Autodesk Fusion 360 part; units mm, degrees
(part 2 of 2)
sketch "Esquisse1" plane through (0, 0, 0) normal (0, 0, 1) x (1, 0, 0)
  circle A0 centre (0, 0) radius 40
  circle A1 centre (0, 0) radius 15
  line L0 (6, 3.4641) -> (0, 6.9282)
  line L1 (0, 6.9282) -> (-6, 3.4641)
  line L2 (-6, 3.4641) -> (-6, -3.4641)
  line L3 (-6, -3.4641) -> (0, -6.9282)
  line L4 (0, -6.9282) -> (6, -3.4641)
  line L5 (6, -3.4641) -> (6, 3.4641)
  circle A2 centre (40, 0) radius 5
  circle A3 centre (0, 0) radius 4.05
  dimension "d21" = 80
  dimension "d26" = 30
  dimension "d27" = 6
  dimension "d122" = 8.1
  constraint coincident A0.centre A1.centre
  constraint concentric A0 A1
  constraint coincident A0 A2.centre
  constraint concentric A1 A3
  measures "d21" diameter of A0
  measures "d26" diameter of A1
  measures "d27" distance of A0.centre L0
  measures "d122" diameter of A3
extrude "Extrusion1" add sketch "Esquisse1" along normal blind 6 contours A0 A2 picked at (28.6857, 8.6025)
extrude "Extrusion2" add sketch "Esquisse1" along normal blind 12 contours A1
extrude "Extrusion3" add sketch "Esquisse1" along normal blind 8 contours L0 L1 L2 L3 L4 L5
pattern_circular "Réseau C1" count 15 over 360 about axis through (0, 0, 0) along (0, 0, 1) of 1 faces at (39.2118, -4.9375, 4)

design "graduation_table_60_Z"
Autodesk Fusion 360 part; units mm, degrees
sketch "Esquisse1" plane through (0, 0, 0) normal (0, 0, 1) x (1, 0, 0)
  arc A0 (169.741, 98) -> (0, 196) centre (0, 0) ccw
  line L0 (0, 182) -> (13, 182)
  line L1 (16, 185) -> (16, 187.4887)
  line L2 (0, 196) -> (0, 193.2049)
  arc A1 (15.7439, 182.0039) -> (15.6111, 182.0119) centre (15.6954, 182.3046) ccw
  arc A2 (19.8621, 190.9699) -> (16, 187.4887) centre (19.5, 187.4887) ccw
  line L3 (0, 0) -> (215.5081, 124.4237) construction
  line L4 (191.1412, 0) -> (248.8473, 0) construction
  line L5 (169.741, 98) -> (157.6166, 91)
  line L6 (157.6166, 91) -> (156.1166, 93.5981)
  line L7 (157.2147, 97.6962) -> (160.0383, 99.3264)
  arc A3 (161.2274, 104.258) -> (19.8621, 190.9699) centre (0, 0) ccw
  line L8 (160.5038, 105.3686) -> (163.9734, 107.3718)
  line L9 (12, 195.6323) -> (12, 191.6246)
  line L10 (1.1843, 192.2221) -> (8, 193.5)
  line L11 (8, 193.5) -> (8, 184.5)
  line L12 (8, 184.5) -> (1.1843, 185.7779)
  line L13 (0, 184.7951) -> (0, 182)
  line L14 (0, 189) -> (13, 189) construction
  arc A4 (13, 182) -> (16, 185) centre (13, 185) ccw
  line L15 (0, 0) -> (0, 230) construction
  line L16 (162.5878, 96.3896) -> (168.6492, 85.891) construction
  line L17 (166.1037, 95.9) -> (170.8023, 90.5262)
  line L18 (170.6759, 89.764) -> (164.2817, 86.0724)
  line L19 (163.5585, 86.344) -> (161.2539, 93.1)
  line L20 (12, 195.6323) -> (12, 182)
  arc A5 (0, 193.2049) -> (1.1843, 192.2221) centre (1, 193.2049) ccw
  arc A6 (1.1843, 185.7779) -> (0, 184.7951) centre (1, 184.7951) ccw
  arc A7 (170.6759, 89.764) -> (170.8023, 90.5262) centre (170.4259, 90.1971) ccw
  arc A8 (163.5585, 86.344) -> (164.2817, 86.0724) centre (164.0317, 86.5054) ccw
  arc A9 (160.0383, 99.3264) -> (161.2274, 104.258) centre (158.2883, 102.3575) ccw
  arc A10 (157.2147, 97.6962) -> (156.1166, 93.5981) centre (158.7147, 95.0981) ccw
  point P0 (154.6166, 96.1962)
  point P1 (0, 192)
  point P2 (0, 186)
  point P3 (171.2027, 90.0682)
  point P4 (163.7549, 85.7682)
  dimension "d38" = 196
  dimension "d47" = 16
  dimension "d58" = 30
  dimension "d60" = 6
  dimension "d68" = 11
  dimension "d69" = 192
  dimension "d70" = 12
  dimension "d77" = 7
  dimension "d83" = 6
  dimension "d84" = 9
  dimension "d85" = 8
  dimension "d86" = 3
  dimension "d87" = 60
  dimension "d88" = 7
  dimension "d89" = 14
  dimension "d90" = 14
  dimension "d91" = 8.6
  dimension "d92" = 5.6
  dimension "d93" = 7.6
  dimension "d94" = 1
  dimension "d95" = 0.5
  dimension "d96" = 0.5
  dimension "d97" = 3.5
  dimension "d98" = 3
  dimension "d99" = 3.5
  constraint perpendicular L0 L1
  constraint tangent L0 A1
  constraint tangent L1 A1
  constraint tangent L1 A2
  constraint coincident A0.centre L3.start
  constraint coincident L3 A0.start
  constraint coincident L3 L5.end
  constraint perpendicular L3 L6
  constraint perpendicular L6 L7
  constraint coincident A3 L8.start
  constraint coincident A0 L8.end
  constraint parallel L3 L8
  constraint horizontal L0
  constraint coincident L2 A0.centre
  constraint coincident A0 L9.start
  constraint coincident A3 L9.end
  constraint vertical L9
  constraint coincident L2 P1
  constraint parallel L2 L11
  constraint perpendicular L0 L13
  constraint perpendicular L11 L14
  constraint symmetric L10 L12 L14
  constraint coincident P2 L13
  constraint tangent A2 A3
  constraint tangent L0 A4
  constraint tangent L1 A4
  constraint vertical L15
  constraint perpendicular L3 L16
  constraint coincident L3 L17.start
  constraint parallel L3 L18
  constraint coincident L5 L19.end
  constraint symmetric L16 L17 L19
  constraint coincident L0 L20.end
  constraint perpendicular L0 L20
  constraint coincident L14.start L2
  constraint coincident P1 L10
  constraint tangent L2 A5
  constraint tangent L10 A5
  constraint coincident P2 L12
  constraint coincident L14.start L13
  constraint tangent L12 A6
  constraint tangent L13 A6
  constraint equal A5 A6
  constraint coincident P3 L17
  constraint coincident P3 L18
  constraint tangent L17 A7
  constraint tangent L18 A7
  constraint coincident P4 L19
  constraint coincident P4 L18
  constraint tangent L19 A8
  constraint tangent L18 A8
  constraint tangent A3 A9
  constraint tangent L7 A9
  constraint coincident P0 L7
  constraint coincident P0 L6
  constraint tangent L7 A10
  constraint tangent L6 A10
  measures "d38" radius of A0
  measures "d47" distance of L1 L2
  measures "d58" angle of L3 L4
  measures "d60" distance of L5.end P0
  measures "d68" distance of L5 L8
  measures "d69" radius of A3
  measures "d70" distance of L2 L9
  measures "d77" distance of A0.end L14.start
  measures "d83" distance of P1 P2
  measures "d84" distance of L10.end L11.end
  measures "d85" distance of L11 L13
  measures "d86" radius of A4
  measures "d87" angle of L3 L15
  measures "d88" distance of A0.start L16
  measures "d89" distance of A0.end L0.start
  measures "d90" distance of A0.start L5.end
  measures "d91" distance of P3 P4
  measures "d92" distance of L17.start L19.end
  measures "d93" distance of L3 L18
  measures "d94" radius of A5
  measures "d95" radius of A7
  measures "d96" radius of A8
  measures "d97" radius of A9
  measures "d98" radius of A10
  measures "d99" radius of A2
extrude "Extrusion4" add sketch "Esquisse1" along normal blind 1.5
sketch "Esquisse3" plane through (0, 0, 0) normal (0, 0, 1) x (-1, 0, 0)
  arc A0 (-169.741, -98) -> (0, -196) centre (0, 0) ccw
  line L0 (0, -196) -> (0, -193.2049)
  line L1 (0, -182) -> (-13, -182)
  line L2 (-16, -185) -> (-16, -187.4887)
  arc A1 (-19.8621, -190.9699) -> (-16, -187.4887) centre (-19.5, -187.4887) ccw
  arc A2 (-161.2274, -104.258) -> (-19.8621, -190.9699) centre (0, 0) ccw
  line L3 (0, 0) -> (-241.9866, 0.0685) construction
  line L4 (0, 0) -> (-178.5811, -129.7468) construction
  line L5 (-160.0383, -99.3264) -> (-157.2147, -97.6962)
  line L6 (-156.1166, -93.5981) -> (-157.6166, -91)
  line L7 (-157.6166, -91) -> (-161.2539, -93.1)
  line L8 (-20, 0) -> (-2.5, 0)
  line L9 (0, 0) -> (-199.6591, -119.8904) construction
  line L10 (0, 0) -> (233.2381, 0) construction
  line L11 (-167.9476, -100.8484) -> (-164.6816, -100.8484)
  line L12 (-164.6816, -100.8484) -> (-166.4127, -97.9656)
  line L13 (-166.4127, -97.9656) -> (-167.9476, -100.8484)
  line L14 (-158.4864, -115.1471) -> (-157.0836, -110.613)
  line L15 (-157.0836, -110.613) -> (-153.7407, -115.2141)
  line L16 (-153.7407, -115.2141) -> (-158.4864, -115.1471)
  line L17 (0, 0) -> (-148.8189, -154.0192) construction
  line L18 (0, 0) -> (214.1862, 0) construction
  line L19 (-1.1843, -192.2221) -> (-8, -193.5)
  line L20 (-8, -193.5) -> (-8, -184.5)
  line L21 (-8, -184.5) -> (-1.1843, -185.7779)
  line L22 (0, -184.7951) -> (0, -182)
  arc A3 (-13, -182) -> (-16, -185) centre (-13, -185) ccw
  line L23 (-161.2539, -93.1) -> (-163.5585, -86.344)
  line L24 (-164.2817, -86.0724) -> (-170.6759, -89.764)
  line L25 (-170.8023, -90.5262) -> (-166.1037, -95.9)
  line L26 (-166.1037, -95.9) -> (-169.741, -98)
  arc A4 (0, -193.2049) -> (-1.1843, -192.2221) centre (-1, -193.2049) ccw
  arc A5 (-1.1843, -185.7779) -> (0, -184.7951) centre (-1, -184.7951) ccw
  arc A6 (-160.0383, -99.3264) -> (-161.2274, -104.258) centre (-158.2883, -102.3575) ccw
  arc A7 (-163.5585, -86.344) -> (-164.2817, -86.0724) centre (-164.0317, -86.5054) ccw
  arc A8 (-170.6759, -89.764) -> (-170.8023, -90.5262) centre (-170.4259, -90.1971) ccw
  arc A9 (-157.2147, -97.6962) -> (-156.1166, -93.5981) centre (-158.7147, -95.0981) ccw
  dimension "d62" = 36
  dimension "d64" = 31
  dimension "d66" = 46
  dimension "d79" = 195.9
  dimension "d80" = 195.9
  dimension "d81" = 3.8
  dimension "d82" = 2.8
  constraint coincident A0.centre A2.centre
  constraint horizontal L10
  constraint horizontal L11
  constraint perpendicular L9 L12
  constraint perpendicular L4 L15
  constraint horizontal L18
  constraint coincident L4 L14.start
  constraint symmetric L4 L14 L16
  constraint coincident L9 L11.start
  constraint symmetric L9 L11 L13
  measures "d62" angle of L4 L8
  measures "d64" angle of L3 L9
  measures "d66" angle of L3 L17
  measures "d79" distance of A0.centre L14.start
  measures "d80" distance of A0.centre L11.start
  measures "d81" distance of L15 L14.start
  measures "d82" distance of L12 L11.start
extrude "Extrusion6" add sketch "Esquisse3" along normal blind 2 contours L11 L12 L13 | L14 L15 L16
pattern_circular "Réseau C4" count 6 over 50 about axis through (0, 0, 0) along (0, 0, 1) of "Extrusion6"
extrude "Extrusion7" add sketch "Esquisse1" along normal blind 2.4 contours A0 L5 L6 L7 A3 L8 A9 A10 | L5 L17 L18 L19 A7 A8 | A0 L0 L2 L9 L10 L11 L12 L13 L20 A5 A6
extrude "Extrusion8" add sketch "Esquisse3" along normal blind 2 contours L11 L12 L13
chamfer "Chanfrein1" distance 0.5 angle 45 1 edges at (162.2386, 106.3702, 2.4)
chamfer "Chanfrein2" distance 0.5 angle 45 2 edges at (12, 188.8162, 2.4) (12, 188.8162, 2.4)
equation "d38 = rayon_externe"
equation "d69 = rayon_externe - 4 mm"
equation "rayon_externe = 196 mm"
equation "d79 = rayon_externe - 0.1 mm"
equation "d80 = rayon_externe - 0.1 mm"
